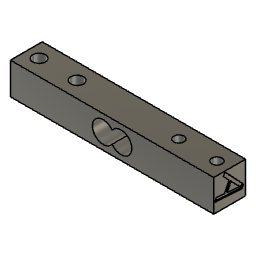
3D Model (Autodesk Fusion 360 archive; units mm, degrees)
design "loadcell design"
Autodesk Fusion 360 part; units mm, degrees
sketch "Sketch1" plane through (0, 0, 0) normal (0, 0, 1) x (1, 0, 0)
  line L0 (40, 6.25) -> (-40, 6.25)
  line L1 (-40, 6.25) -> (-40, -6.25)
  line L2 (-40, -6.25) -> (40, -6.25)
  line L3 (40, -6.25) -> (40, 6.25)
  line L4 (40, 6.25) -> (-40, -6.25) construction
  line L5 (-40, 6.25) -> (40, -6.25) construction
  line L6 (-40, 0) -> (40, 0) construction
  circle A0 centre (-35, 0) radius 2.5
  circle A1 centre (-20, 0) radius 2.5
  circle A2 centre (35, 0) radius 2
  circle A3 centre (20, 0) radius 2
  dimension "d1" = 80
  dimension "d2" = 12.5
  dimension "d3" = 5
  dimension "d4" = 5
  dimension "d5" = 4
  dimension "d6" = 4
  dimension "d7" = 15
  dimension "d8" = 15
  dimension "d9" = 3
  dimension "d10" = 40
  constraint horizontal L0
  constraint perpendicular L0 L1
  constraint parallel L0 L2
  constraint parallel L1 L3
  constraint coincident L4 origin
  constraint coincident L5 origin
  constraint midpoint L1 L6.start
  constraint midpoint L3 L6.end
  constraint coincident L6 A0.centre
  constraint coincident L6 A1.centre
  constraint coincident L6 A2.centre
  constraint coincident L6 A3.centre
  measures "d1" distance of L1.end L2.end
  measures "d2" distance of L0.end L1.end
  measures "d3" diameter of A0
  measures "d4" diameter of A1
  measures "d5" diameter of A2
  measures "d6" diameter of A3
  measures "d7" distance of A2.centre A3.centre
  measures "d8" distance of A0.centre A1.centre
  measures "d9" distance of L3 A2
  measures "d10" distance of A1.centre A3.centre
extrude "Extrude1" add sketch "Sketch1" along normal blind 12.5
sketch "Sketch2" plane through (0, 6.25, 0) normal (0, 1, 0) x (-1, 0, 0)
  line L0 (-40, 0) -> (40, 0)
  line L1 (40, 0) -> (40, 12.5)
  line L2 (40, 12.5) -> (-40, 12.5)
  line L3 (-40, 12.5) -> (-40, 0)
  line L4 (40, 6.25) -> (-40, 6.25) construction
  circle A0 centre (3.5, 6.25) radius 4.25
  circle A1 centre (-3.5, 6.25) radius 4.25
  line L5 (-3.5, 6.25) -> (0, 12.5) construction
  line L6 (3.5, 6.25) -> (0, 12.5) construction
  dimension "d13" = 8.5
  dimension "d14" = 8.5
  dimension "d15" = 15.5
  constraint midpoint L1 L4.start
  constraint midpoint L3 L4.end
  constraint coincident L4 A0.centre
  constraint coincident L4 A1.centre
  constraint coincident A1.centre L5.start
  constraint midpoint L2 L5.end
  constraint coincident A0.centre L6.start
  constraint equal L5 L6
  measures "d13" diameter of A1
  measures "d14" diameter of A0
extrude "Extrude2" cut sketch "Sketch2" against normal blind 24 contours A0 A1 | A0 A1 | A0 A1
sketch "Sketch3" plane through (40, 0, 0) normal (1, 0, 0) x (0, 1, 0)
  line L0 (-6.25, 0) -> (6.25, 0)
  line L1 (6.25, 0) -> (6.25, 12.5)
  line L2 (6.25, 12.5) -> (-6.25, 12.5)
  line L3 (-6.25, 12.5) -> (-6.25, 0)
  line L4 (7.3315, 7.7408) -> (5.9537, 4.8874) construction
  line L5 (5.9537, 4.8874) -> (8.1248, 3.8391) construction
  line L6 (8.1248, 3.8391) -> (9.5026, 6.6926) construction
  line L7 (9.5026, 6.6926) -> (7.3315, 7.7408) construction
  line L8 (6.25, 3.8391) -> (-6.25, 3.8391)
  dimension "d18" = 10
  text T0 "A" font "Arial" height 10 align left top in box 3.1687 x 2.4109 at (7.3315, 7.7408) x (-0.434804, -0.900525) y (0.900525, -0.434804) spacing 1 kerned
  constraint coincident L8
emboss "Emboss1" depth -0.5 profiles "Sketch3" section 1 text T0 onto face at (40, -2.0833, 4.1667)
